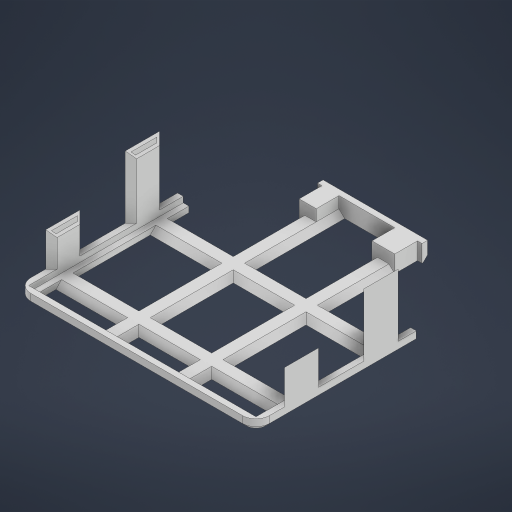
# Autodesk Inventor part: botom_insert
Saved by Autodesk Inventor 2024 (Build 280153000, 153)
## iProperties
Created: 2024-03-20
Part Number: botom_insert
Material: Všeobecné
Document SubType Name: Modeling
Designer: Simak
Density: 1 g/cm^3
Appearance: Výchozí
Author: Simak
Autodesk Inventor part; units mm, degrees
ref_plane "YZ Plane" through (0, 0, 0) normal (1, 0, 0) x (0, 1, 0)
ref_plane "XZ Plane" through (0, 0, 0) normal (0, 1, 0) x (-1, 0, 0)
ref_plane "XY Plane" through (0, 0, 0) normal (0, 0, 1) x (1, 0, 0)
sketch "Náčrt1" plane through (0, 0, 0) normal (0, 1, 0) x (-1, 0, 0)
  line L0 (50, -50) -> (-50, -50)
  line L1 (-50, -50) -> (-50, 50)
  line L2 (-50, 50) -> (50, 50)
  line L3 (50, 50) -> (50, -50)
  line L4 (50, -50) -> (0, 0) construction
  line L5 (0, 0) -> (-50, -50) construction
  line L6 (0, 0) -> (-50, 50) construction
  line L7 (-47.5, -47.5) -> (47.5, -47.5)
  line L8 (47.5, -47.5) -> (47.5, 47.5)
  line L9 (47.5, 47.5) -> (-47.5, 47.5)
  line L10 (-47.5, 47.5) -> (-47.5, -47.5)
  line L11 (-52.5, -52.5) -> (52.5, -52.5)
  line L12 (52.5, -52.5) -> (52.5, 52.5)
  line L13 (52.5, 52.5) -> (-52.5, 52.5)
  line L14 (-52.5, 52.5) -> (-52.5, -52.5)
  line L15 (-47.5, -18) -> (-52.5, -18)
  line L16 (47.5, -18) -> (52.5, -18)
  line L17 (23, -52.5) -> (23, -18)
  line L18 (23, -18) -> (47.5, -18)
  line L19 (-47.5, -18) -> (-23, -18)
  line L20 (-23, -18) -> (-23, -52.5)
  point P0 (-23, -47.5)
  point P1 (-23, -50)
  point P2 (23, -50)
  point P3 (23, -47.5)
  point P4 (-50, -18)
  point P5 (50, -18)
  dimension "d0" = 100
  dimension "d1" = 2.5
  dimension "d2" = 2.5
  dimension "d3" = 68
  dimension "d4" = 27
  dimension "d5" = 27
  constraints: 42 end point, 10 equal length, 8 perpendicular, 7 point on line, 1 collinear, 1 horizontal, 6 other
  measures "d0" distance of L0.start L0.end
  measures "d1" distance between parallel lines of L0 L7
  measures "d2" distance between parallel lines of L0 L11
  measures "d3" distance between parallel lines of L15 L2
  measures "d4" distance between parallel lines of L1 L20
  measures "d5" distance between parallel lines of L3 L17
extrude "Vysunutí1" add sketch "Náčrt1" along normal blind 2.5 contours L0 L20 L7 L17 | L16 L8 L9 L10 L15 L1 L2 L3
extrude "Vysunutí2" add sketch "Náčrt1" along normal blind 5 contours L17 L11 L20 L0 | L3 L2 L1 L15 L14 L13 L12 L16
sketch "Náčrt2" plane through (-23, 0, -47.5) normal (0, 0, 1) x (1, 0, 0)
  line L0 (46, 2.5) -> (0, 2.5) projected
  line L1 (46, 0) -> (0, 0) projected
  line L2 (2, 0) -> (4.5, 2.5)
  line L3 (12, 0) -> (9.5, 2.5)
  line L4 (34, 0) -> (36.5, 2.5)
  line L5 (41.5, 2.5) -> (44, 0)
  line L6 (4.5, 2.5) -> (9.5, 2.5)
  line L7 (12, 0) -> (2, 0)
  line L8 (9.1893, 1.75) -> (10.1893, 0.75)
  line L9 (10.1893, 0.75) -> (3.8107, 0.75)
  line L10 (3.8107, 0.75) -> (4.8107, 1.75)
  line L11 (4.8107, 1.75) -> (9.1893, 1.75)
  line L12 (34, 0) -> (44, 0)
  line L13 (36.5, 2.5) -> (41.5, 2.5)
  line L14 (42.1893, 0.75) -> (41.1893, 1.75)
  line L15 (41.1893, 1.75) -> (36.8107, 1.75)
  line L16 (36.8107, 1.75) -> (35.8107, 0.75)
  line L17 (35.8107, 0.75) -> (42.1893, 0.75)
  point P0 (23, 0)
  dimension "d10" = 45
  dimension "d11" = 2
  dimension "d12" = 2
  dimension "d13" = 5
  dimension "d14" = 5
  dimension "d15" = 0.75
  dimension "d16" = 0.75
  constraints: 32 end point, 8 point on line, 4 collinear, 2 perpendicular, 1 parallel, 6 other
  measures "d10" angle of L1 L2
  measures "d11" distance of L1.end L2.start
  measures "d12" distance of L1.start L5.end
  measures "d13" distance of L3.end L2.end
  measures "d14" distance of L5.start L4.end
  measures "d15" distance between parallel lines of L3 L8
  measures "d16" distance between parallel lines of L5 L14
extrude "Vysunutí3" add sketch "Náčrt2" along normal up to next contours L5 L1 L4 L0 | L3 L1 L2 L0
sketch "Náčrt3" plane through (-47.5, 0, 47.5) normal (1, 0, 0) x (0, 0, -1)
  line L0 (65.5, 2.5) -> (-2.5, 2.5) projected
  line L1 (65.5, 0) -> (-5, 0) projected
  line L2 (0, 0) -> (0, 2.5) projected
  line L3 (65.5, 0) -> (65.5, 2.5) projected
  line L4 (7, 0) -> (9.5, 2.5)
  line L5 (14.5, 2.5) -> (17, 0)
  line L6 (48.5, 0) -> (51, 2.5)
  line L7 (56, 2.5) -> (58.5, 0)
  line L8 (9.5, 2.5) -> (14.5, 2.5)
  line L9 (17, 0) -> (7, 0)
  line L10 (51, 2.5) -> (56, 2.5)
  line L11 (58.5, 0) -> (48.5, 0)
  line L12 (15.1893, 0.75) -> (14.1893, 1.75)
  line L13 (14.1893, 1.75) -> (9.8107, 1.75)
  line L14 (9.8107, 1.75) -> (8.8107, 0.75)
  line L15 (8.8107, 0.75) -> (15.1893, 0.75)
  line L16 (56.6893, 0.75) -> (55.6893, 1.75)
  line L17 (55.6893, 1.75) -> (51.3107, 1.75)
  line L18 (51.3107, 1.75) -> (50.3107, 0.75)
  line L19 (50.3107, 0.75) -> (56.6893, 0.75)
  point P0 (47.5, 0)
  dimension "d19" = 45
  dimension "d20" = 5
  dimension "d21" = 7
  dimension "d22" = 5
  dimension "d23" = 7
  dimension "d24" = 0.75
  dimension "d25" = 0.75
  constraints: 32 end point, 8 point on line, 4 collinear, 2 equal length, 2 perpendicular, 6 other
  measures "d19" angle of L1 L4
  measures "d20" distance of L5.start L4.end
  measures "d21" distance of L2.start L4.start
  measures "d22" distance of L7.start L6.end
  measures "d23" distance of L1.start L7.end
  measures "d24" distance between parallel lines of L5 L12
  measures "d25" distance between parallel lines of L7 L16
extrude "Vysunutí4" add sketch "Náčrt3" along normal up to surface (95 mm away) contours L7 L1 L6 L0 | L5 L1 L4 L0
extrude "Vysunutí5" cut sketch "Náčrt3" along normal up to surface (95 mm away) contours L15 L14 L13 L12 | L19 L18 L17 L16
extrude "Vysunutí6" cut sketch "Náčrt2" along normal up to surface (95 mm away) contours L8 L9 L10 L11 | L17 L16 L15 L14
sketch "Náčrt4" plane through (23, 0, -47.5) normal (1, 0, 0) x (0, 0, -1)
  line L0 (-97.5, 2.5) -> (-29.5, 2.5) projected
  line L1 (0, 2.5) -> (-39, 2.5) projected
  line L2 (2.5, 2.5) -> (0, 2.5) projected
  line L3 (-7.5, 2.5) -> (-7.5, 7.5)
  line L4 (-7.5, 7.5) -> (5, 7.5)
  line L5 (5, 7.5) -> (5, 5)
  line L6 (5, 0) -> (0, 0) projected
  line L7 (0, 0) -> (0, 2.5) projected
  line L8 (2.5, 2.5) -> (0, 2.5) projected
  line L9 (2.5, 2.5) -> (2.5, 5) projected
  line L10 (5, 5) -> (2.5, 5) projected
  line L11 (5, 0) -> (5, 5) projected
  line L12 (-7.5, 2.5) -> (-7.5, 0)
  line L13 (0, 1.75) -> (-39.3107, 1.75) projected
  line L14 (0, 0) -> (-36.5, 0) projected
  point P0 (-47.5, 0)
  dimension "d32" = 90
  dimension "d33" = 5
  constraints: 8 end point, 2 perpendicular, 1 horizontal, 1 point on line, 1 vertical
  measures "d32" distance from line of L0.start L3
  measures "d33" distance from line of L1 L3.end
extrude "Vysunutí7" add sketch "Náčrt4" against normal up to surface (46 mm away) contours L7 L13 L12 L1 | L1 L3 L4 L5 L10 L9 L2 | L7 L14 L12 L13
sketch "Náčrt5" plane through (23, 0, -40) normal (0, 0, 1) x (1, 0, 0)
  line L0 (-2, 0) -> (-4.5, 2.5) projected
  line L1 (0, 0) -> (-2, 0) projected
  line L2 (0, 7.5) -> (0, 0) projected
  line L3 (0, 7.5) -> (-46, 7.5) projected
  line L4 (-46, 7.5) -> (-46, 0) projected
  line L5 (-44, 0) -> (-46, 0) projected
  line L6 (-41.5, 2.5) -> (-44, 0) projected
  line L7 (-36.5, 2.5) -> (-41.5, 2.5) projected
  line L8 (-34, 0) -> (-36.5, 2.5) projected
  line L9 (-12, 0) -> (-34, 0) projected
  line L10 (-9.5, 2.5) -> (-12, 0) projected
  line L11 (-4.5, 2.5) -> (-9.5, 2.5) projected
  line L12 (-2, 0) -> (-2, 7.5)
  line L13 (-12, 0) -> (-12, 7.5)
  line L14 (-34, 0) -> (-34, 7.5)
  line L15 (0, 7.5) -> (-46, 7.5) projected
  line L16 (-44, 0) -> (-44, 7.5)
  line L17 (-36.5, 2.5) -> (-36.5, 7.5)
  point P0 (-23, 0)
  constraints: 10 end point, 5 point on line, 3 perpendicular, 2 parallel
extrude "Vysunutí8" cut sketch "Náčrt5" against normal blind 10 contours L12 L3 L2 L1 | L13 L9 L14 L3 | L14 L8 L17 L3 | L16 L5 L4 L3
fillet "Zaoblení1" radius 6 2 edges at (52.5, 2.5, 52.5) (-52.5, 2.5, 52.5)
chamfer "Zkosení1" distance 2 angle 45 6 edges at (52.5, 0, 14.25) (50.7426, 0, 50.7426) (0, 0, 52.5) (-50.7426, 0, 50.7426) (-52.5, 0, 14.25) (0, 0, -52.5)
sketch "Náčrt6" plane through (0, 5, 0) normal (0, 1, 0) x (1, 0, 0)
  arc A0 (-52.5, -46.5) -> (-46.5, -52.5) centre (-46.5, -46.5) ccw projected
  line L0 (-46.5, -52.5) -> (46.5, -52.5) projected
  arc A1 (46.5, -52.5) -> (52.5, -46.5) centre (46.5, -46.5) ccw projected
  line L1 (52.5, -46.5) -> (52.5, 18) projected
  line L2 (52.5, 18) -> (50, 18) projected
  line L3 (50, 18) -> (50, -50) projected
  line L4 (50, -50) -> (-50, -50) projected
  line L5 (-50, -50) -> (-50, 18) projected
  line L6 (-50, 18) -> (-52.5, 18) projected
  line L7 (-52.5, 18) -> (-52.5, -46.5) projected
  line L8 (-52.5, 10) -> (-50, 7.5)
  line L9 (-50, -2.5) -> (-52.5, -5)
  line L10 (0, -50) -> (0, 0)
  line L11 (-52.5, 18) -> (-52.5, -46.5) projected
  line L12 (-52.5, -25) -> (-50, -27.5)
  line L13 (-50, -37.5) -> (-52.5, -40)
  line L14 (-50, -37.5) -> (-50, -27.5)
  line L15 (-52.5, -25) -> (-52.5, -40)
  line L16 (-50, -2.5) -> (-50, 7.5)
  line L17 (-50, 18) -> (-50, -50) projected
  line L18 (-52.5, 10) -> (-52.5, -5)
  line L19 (-51.75, -38.1893) -> (-50.75, -37.1893)
  line L20 (-50.75, -37.1893) -> (-50.75, -27.8107)
  line L21 (-50.75, -27.8107) -> (-51.75, -26.8107)
  line L22 (-51.75, -26.8107) -> (-51.75, -38.1893)
  line L23 (-51.75, -3.1893) -> (-50.75, -2.1893)
  line L24 (-50.75, -2.1893) -> (-50.75, 7.1893)
  line L25 (-50.75, 7.1893) -> (-51.75, 8.1893)
  line L26 (-51.75, 8.1893) -> (-51.75, -3.1893)
  line L27 (50, -50) -> (50, 18)
  line L28 (52.5, 10) -> (50, 7.5)
  line L29 (50, -2.5) -> (52.5, -5)
  line L30 (52.5, 18) -> (52.5, -46.5)
  line L31 (52.5, -25) -> (50, -27.5)
  line L32 (50, -37.5) -> (52.5, -40)
  line L33 (50, -37.5) -> (50, -27.5)
  line L34 (52.5, -25) -> (52.5, -40)
  line L35 (50, -2.5) -> (50, 7.5)
  line L36 (50, 18) -> (50, -50)
  line L37 (52.5, 10) -> (52.5, -5)
  line L38 (51.75, -38.1893) -> (50.75, -37.1893)
  line L39 (50.75, -37.1893) -> (50.75, -27.8107)
  line L40 (50.75, -27.8107) -> (51.75, -26.8107)
  line L41 (51.75, -26.8107) -> (51.75, -38.1893)
  line L42 (51.75, -3.1893) -> (50.75, -2.1893)
  line L43 (50.75, -2.1893) -> (50.75, 7.1893)
  line L44 (50.75, 7.1893) -> (51.75, 8.1893)
  line L45 (51.75, 8.1893) -> (51.75, -3.1893)
  dimension "d42" = 60
  dimension "d43" = 45
  dimension "d44" = 15
  dimension "d45" = 45
  dimension "d46" = 15
  dimension "d47" = 10
  dimension "d48" = 0.75
  dimension "d49" = 0.75
  constraints: 72 end point, 16 symmetric about line, 13 point on line, 3 collinear, 3 perpendicular, 2 parallel, 1 midpoint, 1 vertical, 6 other
  measures "d42" distance from line of L8.start L4
  measures "d43" angle of L7 L8
  measures "d44" distance of L8.start L9.end
  measures "d45" angle of L7 L12
  measures "d46" distance of L12.start L13.end
  measures "d47" distance from line of L4 L13.end
  measures "d48" distance between parallel lines of L13 L19
  measures "d49" distance between parallel lines of L9 L23
extrude "Vysunutí9" add sketch "Náčrt6" along normal blind 27.5 contours L7 L8 L5 L9 | L29 L3 L28 L1
extrude "Vysunutí10" add sketch "Náčrt6" along normal blind 15 contours L7 L12 L5 L13 | L32 L3 L31 L1
sketch "Náčrt7" plane through (-46.5, 5, 52.5) normal (0, 0, 1) x (1, 0, 0)
  line L0 (-3.5, 0) -> (-6, 0) projected
  line L1 (-3.5, 0) -> (-3.5, 15) projected
  line L2 (-6, 15) -> (-3.5, 15) projected
  line L3 (-6, 0) -> (-6, 15) projected
  line L4 (99, 0) -> (96.5, 0) projected
  line L5 (99, 0) -> (99, 15) projected
  line L6 (96.5, 15) -> (99, 15) projected
  line L7 (96.5, 0) -> (96.5, 15) projected
  line L8 (99, 15) -> (96.5, 12.0206)
  line L9 (-6, 15) -> (-3.5, 12.0206)
  point P0 (46.5, -5)
  dimension "d54" = 50
  dimension "d55" = 50
  constraints: 4 end point, 2 point on line
  measures "d54" angle of L2 L9
  measures "d55" angle of L6 L8
extrude "Vysunutí11" cut sketch "Náčrt7" against normal blind 31 contours L9 L2 L1 | L8 L7 L6
sketch "Náčrt8" plane through (-46.5, 5, 52.5) normal (0, 0, 1) x (1, 0, 0)
  line L0 (-3.5, 0) -> (-6, 0) projected
  line L1 (-3.5, 0) -> (-3.5, 27.5) projected
  line L2 (-6, 27.5) -> (-3.5, 27.5) projected
  line L3 (-6, 0) -> (-6, 27.5) projected
  line L4 (99, 0) -> (96.5, 0) projected
  line L5 (99, 0) -> (99, 27.5) projected
  line L6 (96.5, 27.5) -> (99, 27.5) projected
  line L7 (96.5, 0) -> (96.5, 27.5) projected
  line L8 (99, 27.5) -> (96.5, 24.5206)
  line L9 (96.5, 0) -> (96.5, 27.5) projected
  line L10 (-6, 27.5) -> (-3.5, 24.5206)
  point P0 (46.5, -5)
  dimension "d58" = 40
  constraints: 4 end point, 2 point on line, 1 equal length
  measures "d58" angle of L3 L10
extrude "Vysunutí12" cut sketch "Náčrt8" against normal through all contours L10 L2 L1 | L8 L7 L6
equation "\"d12\" = d11"
equation "\"d14\" = d13"
equation "\"d16\" = d15"
equation "\"d23\" = d21"
equation "\"d25\" = d24"
equation "\"d46\" = d44"
equation "\"d55\" = d54"
